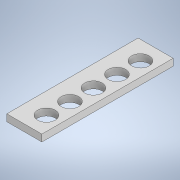
# Autodesk Inventor part: Support
Saved by Autodesk Inventor 2020 (Build 240168000, 168)
## iProperties
Created: 2019-11-07
Part Number: Support
Material: Générique
Document SubType Name: Modeling
Designer: erwan
Density: 1 g/cm^3
Appearance: Par défaut
Author: erwan
Autodesk Inventor part; units mm, degrees
ref_plane "YZ Plane" through (0, 0, 0) normal (1, 0, 0) x (0, 1, 0)
ref_plane "XZ Plane" through (0, 0, 0) normal (0, 1, 0) x (-1, 0, 0)
ref_plane "XY Plane" through (0, 0, 0) normal (0, 0, 1) x (1, 0, 0)
sketch "Esquisse1" plane through (0, 0, 0) normal (0, 1, 0) x (-1, 0, 0)
  line L0 (0, 0) -> (112, 0)
  line L1 (112, 0) -> (112, -419)
  line L2 (112, -419) -> (0, -419)
  line L3 (0, -419) -> (0, 0)
  line L4 (0, -419) -> (45, -419)
  circle A0 centre (45, -59.5) radius 28
  circle A1 centre (45, -134.5) radius 28
  circle A2 centre (45, -209.5) radius 28
  circle A3 centre (45, -284.5) radius 28
  circle A4 centre (45, -359.5) radius 28
  dimension "d0" = 112
  dimension "d1" = 419
  dimension "d8" = 56
  dimension "d9" = 56
  dimension "d10" = 56
  dimension "d11" = 56
  dimension "d12" = 56
  constraints: 10 end point, 5 centre point, 2 parallel, 1 horizontal, 1 perpendicular, 1 point on line
  measures "d0" distance of L1.end L2.end
  measures "d1" distance of L0.end L1.end
  measures "d8" diameter of A0
  measures "d9" diameter of A1
  measures "d10" diameter of A2
  measures "d11" diameter of A3
  measures "d12" diameter of A4
extrude "Extrusion1" add sketch "Esquisse1" along normal blind 22
